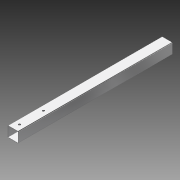
# Autodesk Inventor part: Arm
Saved by Autodesk Inventor 2013 (Build 170138000, 138)
## iProperties
Created: 2011-07-18
Part Number: Arm
Document SubType Name: Modeling
Designer: Nathan
Density: 1 g/cm^3
Material: Generic
Author: Nathan
Autodesk Inventor part; units mm, degrees
ref_plane "YZ Plane" through (0, 0, 0) normal (1, 0, 0) x (0, 1, 0)
ref_plane "XZ Plane" through (0, 0, 0) normal (0, 1, 0) x (-1, 0, 0)
ref_plane "XY Plane" through (0, 0, 0) normal (0, 0, 1) x (1, 0, 0)
sketch "Sketch1" plane through (0, 0, 0) normal (0, 0, 1) x (1, 0, 0)
  line L0 (7.9375, -7.9375) -> (-7.9375, -7.9375)
  line L1 (-7.9375, -7.9375) -> (-7.9375, 7.9375)
  line L2 (-7.9375, 7.9375) -> (7.9375, 7.9375)
  line L3 (7.9375, 7.9375) -> (7.9375, -7.9375)
  line L4 (-7.1437, -7.1438) -> (-7.1437, 7.1437)
  line L5 (-7.1437, 7.1437) -> (7.1437, 7.1438)
  line L6 (7.1437, 7.1438) -> (7.1438, -7.1437)
  line L7 (7.1438, -7.1437) -> (-7.1437, -7.1438)
  line L8 (0, 0) -> (5.5522, 0)
  point P0 (0, 0)
  point P1 (0, 0)
  point P2 (0, 0)
  dimension "d4" = 45
  dimension "d5" = 14.2875
  dimension "d6" = 15.875
  constraints: 18 end point, 3 horizontal, 2 coincident, 1 point on line, 19 other
  measures "d5" distance of L4.start L4.end
  measures "d6" distance of L1.end L2.end
extrude "Extrusion1" add sketch "Sketch1" along normal blind 228.6
sketch "Sketch2" plane through (-7.9375, 7.9375, 0) normal (0, 1, 0) x (1, 0, 0)
  line L0 (0, -228.6) -> (15.875, -228.6) projected
  line L1 (15.875, 0) -> (15.875, -228.6) projected
  line L2 (0, 0) -> (0, -228.6) projected
  line L3 (7.9375, -228.6) -> (7.9375, -257.0929)
  line L4 (7.9375, -219.075) -> (26.9875, -219.075) construction
  point P0 (7.9375, 0)
  point P1 (7.9375, -183.515)
  dimension "d27" = 9.525
  dimension "d30" = 35.56
  constraints: 4 end point, 2 parallel, 2 point on line, 1 horizontal, 1 midpoint
  measures "d27" distance of L3.start L4.start
  measures "d30" distance of point (7.937, -183.515) L4.start
hole "Hole1" at (0, 7.9375, 219.075) at (0, 7.9375, 183.515) direction (0, -1, 0) diameter 3.302 end through all thread size "8-32 UNC" class "2B" standard "ANSI Unified Screw Threads"
fillet "Fillet1" radius 1.27 4 edges at (-7.9375, 7.9375, 114.3) (7.9375, 7.9375, 114.3) (7.9375, -7.9375, 114.3) (-7.9375, -7.9375, 114.3)
body "Solid1"
